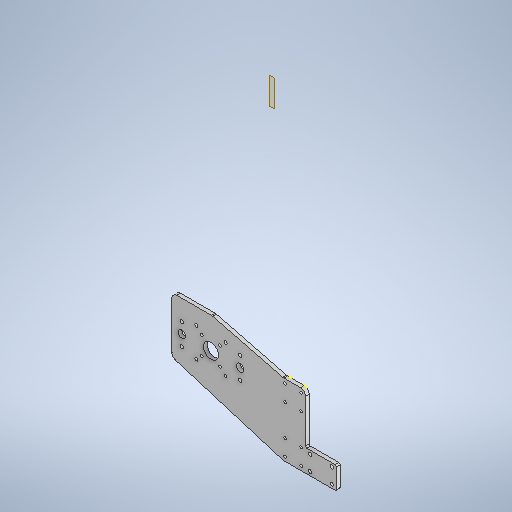
# Autodesk Inventor part: SIDE SUPPORT PLATES
Saved by Autodesk Inventor 2025.2 (Build 292293000, 293)
## iProperties
Created: 2026-02-05
Part Number: SIDE SUPPORT PLATES
Material: Generic
Document SubType Name: Modeling
Designer: composite
Density: 1 g/cm^3
Appearance: Default
Author: composite
Autodesk Inventor part; units mm, degrees
ref_plane "YZ Plane" through (0, 0, 0) normal (1, 0, 0) x (0, 1, 0)
ref_plane "XZ Plane" through (0, 0, 0) normal (0, 1, 0) x (-1, 0, 0)
ref_plane "XY Plane" through (0, 0, 0) normal (0, 0, 1) x (1, 0, 0)
ref_plane "Work Plane1" through (26.2088, 494.2322, 0) normal (0, 0, 1) x (-1, 0, 0)
sketch "Sketch1" plane through (26.2088, 494.2322, 0) normal (0, 0, 1) x (-1, 0, 0)
  line L0 (-27.8436, 404.4322) -> (-27.8436, 443.8322) projected
  line L1 (-27.8436, 404.4322) -> (-20.8436, 404.4322) projected
  line L2 (-20.8436, 404.4322) -> (-20.8436, 443.8322) projected
  line L3 (-27.8436, 443.8322) -> (-20.8436, 443.8322) projected
  arc A0 (-25.8436, 437.1322) -> (-21.8436, 437.1322) centre (-23.8436, 437.1322) ccw projected
  arc A1 (-21.8436, 437.1322) -> (-25.8436, 437.1322) centre (-23.8436, 437.1322) ccw projected
  arc A2 (-25.8436, 411.1322) -> (-21.8436, 411.1322) centre (-23.8436, 411.1322) ccw projected
  arc A3 (-21.8436, 411.1322) -> (-25.8436, 411.1322) centre (-23.8436, 411.1322) ccw projected
  line L4 (-52.8436, 404.4322) -> (-52.8436, 443.8322) projected
  line L5 (-52.8436, 404.4322) -> (-45.8436, 404.4322) projected
  line L6 (-45.8436, 404.4322) -> (-45.8436, 443.8322) projected
  line L7 (-52.8436, 443.8322) -> (-45.8436, 443.8322) projected
  arc A4 (-51.8436, 437.1322) -> (-47.8436, 437.1322) centre (-49.8436, 437.1322) ccw projected
  arc A5 (-47.8436, 437.1322) -> (-51.8436, 437.1322) centre (-49.8436, 437.1322) ccw projected
  arc A6 (-51.8436, 411.1322) -> (-47.8436, 411.1322) centre (-49.8436, 411.1322) ccw projected
  arc A7 (-47.8436, 411.1322) -> (-51.8436, 411.1322) centre (-49.8436, 411.1322) ccw projected
  line L8 (-45.8436, 520.2322) -> (-45.8436, 480.8322) projected
  line L9 (-45.8436, 520.2322) -> (-52.8436, 520.2322) projected
  line L10 (-52.8436, 520.2322) -> (-52.8436, 480.8322) projected
  line L11 (-45.8436, 480.8322) -> (-52.8436, 480.8322) projected
  arc A8 (-47.8436, 487.5322) -> (-51.8436, 487.5322) centre (-49.8436, 487.5322) ccw projected
  arc A9 (-51.8436, 487.5322) -> (-47.8436, 487.5322) centre (-49.8436, 487.5322) ccw projected
  arc A10 (-47.8436, 513.5322) -> (-51.8436, 513.5322) centre (-49.8436, 513.5322) ccw projected
  arc A11 (-51.8436, 513.5322) -> (-47.8436, 513.5322) centre (-49.8436, 513.5322) ccw projected
  line L12 (-20.8436, 520.2322) -> (-20.8436, 480.8322) projected
  line L13 (-20.8436, 520.2322) -> (-27.8436, 520.2322) projected
  line L14 (-27.8436, 520.2322) -> (-27.8436, 480.8322) projected
  line L15 (-20.8436, 480.8322) -> (-27.8436, 480.8322) projected
  arc A12 (-21.8436, 487.5322) -> (-25.8436, 487.5322) centre (-23.8436, 487.5322) ccw projected
  arc A13 (-25.8436, 487.5322) -> (-21.8436, 487.5322) centre (-23.8436, 487.5322) ccw projected
  arc A14 (-21.8436, 513.5322) -> (-25.8436, 513.5322) centre (-23.8436, 513.5322) ccw projected
  arc A15 (-25.8436, 513.5322) -> (-21.8436, 513.5322) centre (-23.8436, 513.5322) ccw projected
sketch "Sketch2" plane through (26.2088, 494.2322, 0) normal (0, 0, 1) x (-1, 0, 0)
  line L0 (-20.8436, 110.4465) -> (-27.8436, 110.4465) projected
  line L1 (10, 520.2322) -> (10, 480.8322) projected
  line L2 (-45.8436, 520.2322) -> (-52.8436, 520.2322) projected
  line L3 (-52.8436, 520.2322) -> (-52.8436, 480.8322) projected
  line L4 (-52.8436, 404.4322) -> (-45.8436, 404.4322) projected
  line L5 (-27.8436, 404.4322) -> (-20.8436, 404.4322) projected
  line L6 (-20.8436, 520.2322) -> (-52.8436, 520.2322)
  line L7 (-52.8436, 404.4322) -> (-20.8436, 404.4322)
  line L8 (159.1564, 465.2322) -> (159.1564, 375.2322)
  line L9 (124.1564, 453.4322) -> (67.7564, 453.4322) construction
  line L10 (67.7564, 453.4322) -> (67.7564, 397.0322) construction
  line L11 (67.7564, 397.0322) -> (124.1564, 397.0322) construction
  line L12 (124.1564, 397.0322) -> (124.1564, 453.4322) construction
  line L13 (159.1564, 375.2322) -> (94.1564, 375.2322)
  line L14 (94.1564, 375.2322) -> (-20.8436, 404.4322)
  line L15 (159.1564, 465.2322) -> (-20.8436, 520.2322)
  circle A0 centre (143.1564, 425.2322) radius 6.025
  circle A1 centre (48.7564, 425.2322) radius 6.025
  circle A2 centre (-23.8436, 513.5322) radius 2.15
  circle A3 centre (-23.8436, 487.5322) radius 2.15
  circle A4 centre (-23.8436, 437.1322) radius 2.15
  circle A5 centre (-23.8436, 411.1322) radius 2.15
  circle A6 centre (-49.8436, 411.1322) radius 2.15
  circle A7 centre (-49.8436, 437.1322) radius 2.15
  circle A8 centre (-49.8436, 487.5322) radius 2.15
  circle A9 centre (-49.8436, 513.5322) radius 2.15
  line L16 (-52.8436, 520.2322) -> (-56.8436, 520.2322)
  line L17 (-56.8436, 520.2322) -> (-56.8436, 404.4322)
  line L18 (-56.8436, 404.4322) -> (-52.8436, 404.4322)
  circle A10 centre (119.5264, 448.8022) radius 2.5
  circle A11 centre (119.5264, 401.6622) radius 2.5
  circle A12 centre (72.3864, 401.6622) radius 2.5
  circle A13 centre (72.3864, 448.8022) radius 2.5
  line L19 (119.5264, 448.8022) -> (119.5264, 401.6622) construction
  line L20 (119.5264, 401.6622) -> (72.3864, 401.6622) construction
  line L21 (119.5264, 448.8022) -> (72.3864, 401.6622) construction
  line L22 (119.5264, 401.6622) -> (72.3864, 448.8022) construction
  circle A14 centre (95.9564, 425.2322) radius 12
  circle A15 centre (143.1564, 442.7322) radius 2.75
  circle A16 centre (143.1564, 407.7322) radius 2.75
  circle A17 centre (48.7564, 407.7322) radius 2.75
  circle A18 centre (48.7564, 442.7322) radius 2.75
  circle A19 centre (110.8056, 410.383) radius 2.25
  circle A20 centre (110.8056, 440.0815) radius 2.25
  circle A21 centre (81.1071, 440.0815) radius 2.25
  circle A22 centre (81.1071, 410.383) radius 2.25
  arc A23 (-25.8436, 487.5322) -> (-21.8436, 487.5322) centre (-23.8436, 487.5322) ccw projected
  arc A24 (-25.8436, 513.5322) -> (-21.8436, 513.5322) centre (-23.8436, 513.5322) ccw projected
  line L23 (-53.8436, 520.2322) -> (-53.8436, 480.8322) projected
  line L24 (-56.8436, 520.2322) -> (-106.8436, 520.2322)
  line L25 (-106.8436, 520.2322) -> (-106.8436, 484.2322)
  line L26 (-106.8436, 484.2322) -> (-56.8436, 484.2322)
  circle A25 centre (-64.3436, 514.2322) radius 2.75
  circle A26 centre (-64.3436, 490.2322) radius 2.75
  circle A27 centre (-99.3436, 490.2322) radius 2.75
  circle A28 centre (-99.3436, 514.2322) radius 2.75
  line L27 (48.7564, 425.2322) -> (-81.8436, 425.2322) construction
  point P0 (26.2088, 494.2322)
  point P1 (-27.8436, 520.2322)
  point P2 (-20.8436, 480.8322)
  point P3 (124.1564, 425.2322)
  point P4 (159.1564, 420.2322)
  point P5 (-27.8436, 520.2322)
  point P6 (119.5264, 425.2322)
  point P7 (95.9564, 401.6622)
  point P8 (95.9564, 397.0322)
  point P9 (95.9564, 425.2322)
  dimension "d1" = 90
  dimension "d2" = 56.4
  dimension "d3" = 56.4
  dimension "d4" = 180
  dimension "d5" = 55
  dimension "d7" = 12.05
  dimension "d9" = 19
  dimension "d10" = 19
  dimension "d12" = 40
  dimension "d13" = 65
  dimension "d14" = 4.3
  dimension "d18" = 4
  dimension "d19" = 5
  dimension "d20" = 47.14
  dimension "d21" = 47.14
  dimension "d22" = 24
  dimension "d23" = 5.5
  dimension "d24" = 35
  dimension "d25" = 17.5
  dimension "d26" = 4.5
  dimension "d27" = 42
  dimension "d28" = 63.2
  dimension "d29" = 36
  dimension "d30" = 24
  dimension "d31" = 35
  dimension "d32" = 5.5
  dimension "d33" = 6
  dimension "d34" = 7.5
  dimension "d35" = 53
  constraints: 42 end point, 27 centre point, 20 equal radius, 11 horizontal alignment, 11 vertical alignment, 8 coincident, 8 horizontal, 7 midpoint, 5 point on line, 4 perpendicular, 2 parallel, 2 vertical, 1 collinear, 1 other
  measures "d1" distance of L8.start L8.end
  measures "d2" distance of L11.end L9.start
  measures "d3" distance of L10.end L11.end
  measures "d4" distance from line of L1.start L8
  measures "d5" vertical distance of L1.start L8.start
  measures "d7" diameter of A0
  measures "d9" distance of point (124.156, 425.232) A0.centre
  measures "d10" distance from line of L10 L27.start
  measures "d12" vertical distance of L8.start A0.centre
  measures "d13" distance of L8.end L13.end
  measures "d14" diameter of A2
  measures "d18" distance from line of L17 L2.end
  measures "d19" diameter of A11
  measures "d20" distance of L20.end L19.end
  measures "d21" distance of L19.end L19.start
  measures "d22" diameter of A14
  measures "d23" diameter of A15
  measures "d24" distance of A16.centre A15.centre
  measures "d25" distance of A18.centre L27.start
  measures "d26" diameter of A19
  measures "d27" distance of A20.centre A22.centre
  measures "d28" distance from line of L8 point (95.956, 425.232)
  measures "d29" distance of L24.end L25.end
  measures "d30" distance of A27.centre A28.centre
  measures "d31" distance of A28.centre A25.centre
  measures "d32" diameter of A25
  measures "d33" distance from line of L24 A28.centre
  measures "d34" distance from line of L25 A28.centre
  measures "d35" distance between parallel lines of L23 L25
extrude "Extrusion1" add sketch "Sketch2" along normal blind 6
fillet "Fillet1" radius 8 6 edges at (-132.9476, 29, 3) (-132.9476, 119, 3) (-67.9476, 119, 3) (47.0524, -26, 3) (47.0524, 89.8, 3) (83.0524, 89.8, 3)
fillet "Fillet2" radius 2 3 edges at (133.0524, -26, 3) (133.0524, 10, 3) (83.0524, 10, 3)
equation "\"d10\" = d9"
equation "\"d25\" = 0.5 * d24"
body "Solid1"
